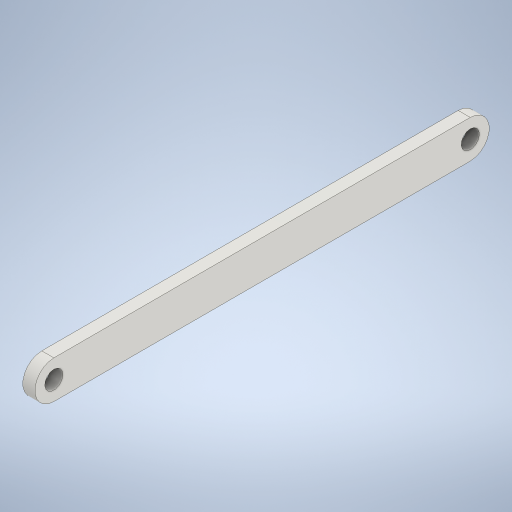
# Autodesk Inventor part: Braço Macaco
Saved by Autodesk Inventor 2024 (Build 280153000, 153)
## iProperties
Created: 2024-06-01
Part Number: Braço Macaco
Material: Steel AISI 4142 380 QT
Document SubType Name: Modeling
Designer: Pedro
Density: 7.85 g/cm^3
Appearance: Steel
Mass: 448.372 g
Surface Area: 199.109 cm^2
Volume: 57.1174 cm^3
Author: Pedro
Autodesk Inventor part; units mm, degrees
ref_plane "YZ Plane" through (0, 0, 0) normal (1, 0, 0) x (0, 1, 0)
ref_plane "XZ Plane" through (0, 0, 0) normal (0, 1, 0) x (-1, 0, 0)
ref_plane "XY Plane" through (0, 0, 0) normal (0, 0, 1) x (1, 0, 0)
sketch "Sketch1" plane through (0, 0, 0) normal (1, 0, 0) x (0, 1, 0)
  line L0 (12.5, 150) -> (12.5, -150)
  line L1 (12.5, -150) -> (-12.5, -150)
  line L2 (-12.5, -150) -> (-12.5, 150)
  line L3 (-12.5, 150) -> (12.5, 150)
  circle A0 centre (0, 137.5) radius 6
  circle A1 centre (0, -137.5) radius 6
  point P0 (0, 0)
  point P1 (-12.5, 56.5)
  point P2 (-12.5, 60.4432)
  dimension "d0" = 300
  dimension "d1" = 25
  dimension "d2" = 12.5
  dimension "d3" = 150
  dimension "d4" = 12
  dimension "d5" = 12.5
  dimension "d6" = 12
  dimension "d7" = 12.5
  constraints: 8 end point, 2 centre point, 2 parallel, 2 point on line, 1 perpendicular, 1 vertical
  measures "d0" distance of L0.start L0.end
  measures "d1" distance of L0.end L1.end
  measures "d2" distance from line of point (0, 0) L0
  measures "d3" distance from line of point (0, 0) L3
  measures "d4" diameter of A0
  measures "d5" distance from line of L3 A0.centre
  measures "d6" diameter of A1
  measures "d7" distance from line of L1 A1.centre
extrude "Extrusion1" add sketch "Sketch1" along normal blind 8
full round fillet "Full Round Fillet1" first side at (2.6667, 12.5, -50) centre faces at (2.6667, 4.1667, 150) second side at (2.6667, -12.5, 50)
full round fillet "Full Round Fillet2" first side at (5.3333, 12.5, -54.1666) centre faces at (2.6667, -4.1667, -150) second side at (5.3333, -12.5, 41.6667)
body "Solid1"
